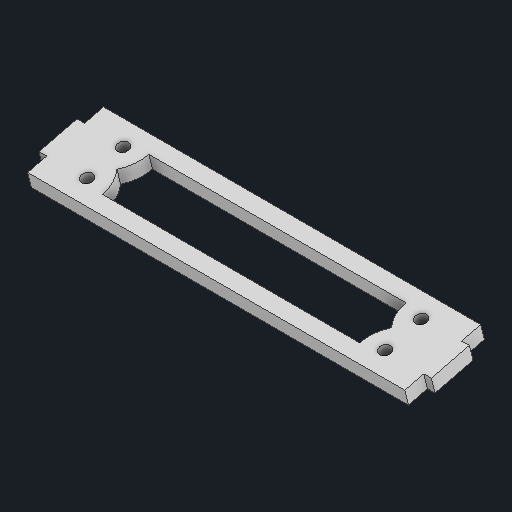
# Autodesk Inventor part: motor_mount
Saved by Autodesk Inventor 2023 (Build 270158030, 158C)
## iProperties
Created: 2022-03-25
Part Number: motor_mount
Material: Generic
Document SubType Name: Modeling
Designer: kardo
Density: 1 g/cm^3
Appearance: Default
Author: kardo
Autodesk Inventor part; units mm, degrees
ref_plane "YZ Plane" through (0, 0, 0) normal (1, 0, 0) x (0, 1, 0)
ref_plane "XZ Plane" through (0, 0, 0) normal (0, 1, 0) x (-1, 0, 0)
ref_plane "XY Plane" through (0, 0, 0) normal (0, 0, 1) x (1, 0, 0)
derived "parameters_frame.ipt"
derived "stencil_frame.ipt"
sketch "sk_cowl_joint_locations" plane through (54.6, 0, 0) normal (1, 0, 0) x (0, 1, 0)
  line L0 (-363, 18.496) -> (-275.8801, 20.463) construction
  arc A0 (-275.8801, 20.463) -> (-254.1001, 21.0191) centre (-359.1231, 3707.4463) ccw construction
  line L1 (-254.1001, 21.0191) -> (9.48, 28.5282) construction
  arc A1 (30.81, 28.832) -> (9.48, 28.5282) centre (30.81, -720.1791) ccw construction
  line L2 (30.81, 28.832) -> (94.8, 28.832) construction
  line L3 (94.8, 30.032) -> (30.81, 30.032) construction
  arc A2 (30.81, 30.032) -> (9.4458, 29.7277) centre (30.81, -720.1791) ccw construction
  line L4 (9.4458, 29.7277) -> (-254.1343, 22.2186) construction
  arc A3 (-275.9072, 21.6626) -> (-254.1343, 22.2186) centre (-359.1231, 3707.4463) ccw construction
  line L5 (-275.9072, 21.6626) -> (-363, 19.6963) construction
  line L6 (-242.0001, 4592.9714) -> (-242.0001, -1605.7041) construction
  line L7 (-120.9999, 4592.9714) -> (-120.9999, -1605.7041) construction
  line L8 (-363, 4592.9714) -> (-363, -1605.7041) construction
  line L9 (0, 4592.9714) -> (0, -1605.7041) construction
  line L10 (-242.0001, 45.0688) -> (-242.0001, 22.5643) construction
  line L11 (-120.9999, 49.9661) -> (-120.9999, 26.0115) construction
  line L12 (-363, 19.6963) -> (-363, 19.6963)
  line L13 (-363, 19.6963) -> (-363, 36.9211) construction
  line L14 (-1229.7832, 4422.8213) -> (280.3081, -1633.8241) construction
  line L15 (-362.7741, 36.9211) -> (-363, 39.712) construction
  line L16 (0, 51.6) -> (0, 29.4586) construction
  line L17 (-142.5135, 45.4866) -> (-137.5404, 25.5402) construction
  line L18 (-134.9025, 31.4945) -> (-138.7836, 30.5268) construction
  line L19 (-137.3891, 41.4677) -> (-141.2702, 40.5) construction
  spline S0 degree 2 poles (-363, 39.712) (-181.6483, 54.394) (0, 54.4) knots 0 0 0 1 1 1
  spline S1 degree 3 poles (0, 54.4) (31.284, 54.4) (68.256, 47.9917) (94.8, 37.536) knots 1 1 1 1 2 2 2 2
  spline S2 degree 3 poles (93.7738, 34.9308) (89.4268, 36.6431) (81.2968, 39.4556) (71.234, 42.2519) (63.4432, 44.1558) (58.1419, 45.3261) (51.4169, 46.6598) (45.9725, 47.6212) (39.1225, 48.6857) (33.6211, 49.4253) (26.7536, 50.2046) (21.2812, 50.7098) (14.5037, 51.1886) (7.8073, 51.5121) (2.5751, 51.6) (0, 51.6) knots 1 1 1 1 1.166667 1.291667 1.333333 1.416667 1.458333 1.541667 1.583333 1.666667 1.708333 1.791667 1.833333 1.916667 2 2 2 2
  spline S3 degree 3 poles (0, 51.6) (-20.1706, 51.5993) (-55.4643, 51.3605) (-95.7903, 50.6123) (-126.0307, 49.8474) (-146.1889, 49.2356) (-171.3841, 48.3435) (-191.5382, 47.528) (-216.7283, 46.3813) (-236.8783, 45.3621) (-262.0632, 43.9608) (-282.2091, 42.7379) (-307.3889, 41.082) (-332.5661, 39.2987) (-352.7052, 37.7363) (-362.7741, 36.9211) knots 0 0 0 0 0.166667 0.291667 0.333333 0.416667 0.458333 0.541667 0.583333 0.666666 0.708333 0.791666 0.833333 0.916666 1 1 1 1
  line L20 (-142.5135, 45.4866) -> (-138.6324, 46.4543) construction
  line L21 (-137.5404, 25.5402) -> (-133.6592, 26.5079) construction
  line L22 (-138.6324, 46.4543) -> (-138.8117, 52.2515) construction
  point P0 (0, 0)
  point P1 (-363, 28.3087)
  point P2 (-242.0001, 33.8165)
  point P3 (-120.9999, 37.9888)
  point P4 (0, 40.5293)
  point P5 (0, 40.5293)
ref_plane "plane_motor_mount" through (0, -127.05, 0) normal (0, 0.9702957, 0.2419219) x (-1, 0, 0)
ref_plane "plane_cowl_right" through (54.6, 0, 0) normal (1, 0, 0) x (0, 1, 0)
ref_plane "plane_symmetry" through (0, 0, 0) normal (1, 0, 0) x (0, 1, 0)
sketch "sk_base" plane through (0, -127.05, 0) normal (0, 0.9702957, 0.2419219) x (-1, 0, 0)
  line L0 (-54.6, -1634.5025) -> (-54.6, 4536.9515) construction
  line L1 (0, -1634.5025) -> (0, 4536.9515) projected
  line L2 (0, 47.8764) -> (-49.6, 47.8764)
  line L3 (-49.6, 47.8764) -> (-49.6, 42.7372)
  line L4 (-49.6, 42.7372) -> (-51.6, 42.7372)
  line L5 (-51.6, 42.7372) -> (-51.6, 32.4587)
  line L6 (-51.6, 32.4587) -> (-49.6, 32.4587)
  line L7 (-49.6, 32.4587) -> (-49.6, 27.3194)
  line L8 (-49.6, 27.3194) -> (0, 27.3194)
  point P0 (0, -30.7362)
  point P1 (-54.6, 42.7372)
  point P2 (-54.6, 32.4587)
  point P3 (-54.6, 47.8764)
  point P4 (-54.6, 27.3194)
  dimension "d2" = 5
  dimension "d3" = 2
  constraints: 14 end point, 6 point on line, 4 perpendicular, 2 parallel, 1 collinear
  measures "d2" distance between parallel lines of L0 L3
  measures "d3" distance between parallel lines of L3 L5
extrude "thicken" add sketch "sk_base" against normal blind 4
sketch "sk_cut" plane through (0, -127.05, 0) normal (0, 0.9702957, 0.2419219) x (-1, 0, 0)
  line L0 (-49.6, 27.3194) -> (0, 27.3194) construction
  line L1 (0, 27.3194) -> (0, 47.8764) projected
  line L2 (0, 47.8764) -> (-49.6, 47.8764) construction
  line L3 (-49.6, 47.8764) -> (-49.6, 42.7372) construction
  line L4 (-49.6, 42.7372) -> (-51.6, 42.7372) construction
  line L5 (-51.6, 42.7372) -> (-51.6, 32.4587) construction
  line L6 (-51.6, 32.4587) -> (-49.6, 32.4587) construction
  line L7 (-49.6, 32.4587) -> (-49.6, 27.3194) construction
  line L8 (0, 27.3194) -> (0, 47.8764) projected
  line L9 (0, 43.8764) -> (-33.8, 43.8764)
  line L10 (0, 31.3194) -> (-33.8, 31.3194)
  arc A0 (-33.8, 31.3194) -> (-36.0852, 37.5979) centre (-43.5676, 31.3194) ccw
  arc A1 (-36.0852, 37.5979) -> (-33.8, 43.8764) centre (-43.5676, 43.8764) ccw
  circle A2 centre (-39.2, 42.4764) radius 1.5
  circle A3 centre (-39.2, 32.7194) radius 1.5
  line L11 (-44.6, 47.8764) -> (-44.6, 27.3194) construction
  line L12 (-33.8, 43.8764) -> (-33.8, 31.3194) construction
  line L13 (-39.2, 32.7194) -> (-44.6, 32.7194) construction
  line L14 (-39.2, 32.7194) -> (-39.2, 27.3194) construction
  line L15 (-39.2, 42.4764) -> (-39.2, 47.8764) construction
  line L16 (-39.2, 42.4764) -> (-44.6, 42.4764) construction
  point P0 (0, -30.7362)
  point P1 (-34.3891, 34.6601)
  dimension "d7" = 3
  dimension "d11" = 4
  dimension "d12" = 4
  dimension "d13" = 140
  dimension "d22" = 5
  dimension "d23" = 5.4
  dimension "d24" = 5.4
  constraints: 16 end point, 9 point on line, 5 point on circle, 4 centre point, 4 perpendicular, 3 equal length, 3 parallel, 2 equal radius, 2 line through centre
  measures "d7" diameter of A2
  measures "d11" distance between parallel lines of L2 L9
  measures "d12" distance between parallel lines of L0 L10
  measures "d22" distance between parallel lines of L11 L3
  measures "d23" distance between parallel lines of L11 L14
  measures "d24" distance between parallel lines of L14 L12
extrude "cut" cut sketch "sk_cut" along normal through all both and the other way through all
mirror "mirror" about plane through (0, 0, 0) normal (1, 0, 0)
equation "\"d2\" = cowl_liner_width"
equation "\"d3\" = bulkhead_thickness"
equation "\"d4\" = 2 * bulkhead_thickness"
equation "\"d7\" = drill_motor_mount_diam"
equation "\"d11\" = bulkhead_inset"
equation "\"d12\" = bulkhead_inset"
equation "\"d22\" = cowl_sealing_width"
equation "\"d23\" = 1.8 * drill_motor_mount_diam"
equation "\"d24\" = 1.8 * drill_motor_mount_diam"
equation "\"cowl_liner_width\" = 5"
equation "\"bulkhead_thickness\" = 2"
equation "\"drill_motor_mount_diam\" = 3"
equation "\"bulkhead_inset\" = 4"
equation "\"cowl_sealing_width\" = 5"
body "Solid1"
